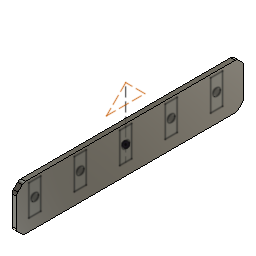
SKADIS_SNS_Label (Autodesk Fusion 360 design; units mm, degrees)
Autodesk Fusion 360 part; units mm, degrees
sketch "SlotLayout" plane through (0, 0, 0) normal (1, 0, 0) x (0, 1, 0)
  line L0 (-22.4, 25) -> (-22.4, 15)
  line L1 (82.4, 5) -> (82.4, -5)
  line L2 (-37.6, -5) -> (-37.6, 5)
  line L3 (-80, 5) -> (-80, -5) construction
  line L4 (-97.6, 15) -> (-97.6, 25)
  line L5 (2.4, -5) -> (2.4, 5)
  arc A0 (-77.6, 5) -> (-82.4, 5) centre (-80, 5) ccw
  arc A1 (22.4, 25) -> (17.6, 25) centre (20, 25) ccw
  arc A2 (-97.6, 25) -> (-102.4, 25) centre (-100, 25) ccw
  arc A3 (97.6, 15) -> (102.4, 15) centre (100, 15) ccw
  line L6 (-60, 25) -> (-60, 15) construction
  line L7 (-77.6, -5) -> (-77.6, 5)
  arc A4 (77.6, -5) -> (82.4, -5) centre (80, -5) ccw
  line L8 (-40, 5) -> (-40, -5) construction
  line L9 (-57.6, 15) -> (-57.6, 25)
  line L10 (-62.4, 25) -> (-62.4, 15)
  line L11 (-102.4, 25) -> (-102.4, 15)
  line L12 (97.6, 15) -> (97.6, 25)
  arc A5 (-102.4, 15) -> (-97.6, 15) centre (-100, 15) ccw
  line L13 (20, 25) -> (20, 15) construction
  line L14 (22.4, 25) -> (22.4, 15)
  line L15 (-80, 0) -> (0, 0) construction
  line L16 (62.4, 25) -> (62.4, 15)
  line L17 (42.4, 5) -> (42.4, -5)
  arc A6 (2.5, 5) -> (-2.5, 5) centre (0, 5) ccw
  arc A7 (2.4, 5) -> (-2.4, 5) centre (0, 5) ccw
  line L18 (80, 5) -> (80, -5) construction
  arc A8 (82.4, 5) -> (77.6, 5) centre (80, 5) ccw
  arc A9 (-2.5, -5) -> (2.5, -5) centre (0, -5) ccw
  arc A10 (57.6, 15) -> (62.4, 15) centre (60, 15) ccw
  arc A11 (62.4, 25) -> (57.6, 25) centre (60, 25) ccw
  line L19 (17.6, 15) -> (17.6, 25)
  line L20 (-20, 25) -> (-20, 15) construction
  line L21 (-42.4, 5) -> (-42.4, -5)
  line L22 (60, 25) -> (60, 15) construction
  arc A12 (42.4, 5) -> (37.6, 5) centre (40, 5) ccw
  line L23 (-100, 25) -> (-100, 15) construction
  line L24 (100, 25) -> (100, 15) construction
  arc A13 (-57.6, 25) -> (-62.4, 25) centre (-60, 25) ccw
  arc A14 (37.6, -5) -> (42.4, -5) centre (40, -5) ccw
  line L25 (40, 5) -> (40, -5) construction
  line L26 (-17.6, 15) -> (-17.6, 25)
  arc A15 (-17.6, 25) -> (-22.4, 25) centre (-20, 25) ccw
  line L27 (-82.4, 5) -> (-82.4, -5)
  line L28 (-2.5, 5) -> (-2.5, -5)
  line L29 (-2.4, 5) -> (-2.4, -5)
  line L30 (102.4, 25) -> (102.4, 15)
  arc A16 (17.6, 15) -> (22.4, 15) centre (20, 15) ccw
  arc A17 (-22.4, 15) -> (-17.6, 15) centre (-20, 15) ccw
  line L31 (37.6, -5) -> (37.6, 5)
  line L32 (0, 5) -> (0, -5) construction
  arc A18 (-62.4, 15) -> (-57.6, 15) centre (-60, 15) ccw
  arc A19 (-42.4, -5) -> (-37.6, -5) centre (-40, -5) ccw
  arc A20 (-2.4, -5) -> (2.4, -5) centre (0, -5) ccw
  arc A21 (102.4, 25) -> (97.6, 25) centre (100, 25) ccw
  arc A22 (-82.4, -5) -> (-77.6, -5) centre (-80, -5) ccw
  arc A23 (-37.6, 5) -> (-42.4, 5) centre (-40, 5) ccw
  line L33 (77.6, -5) -> (77.6, 5)
  line L34 (57.6, 15) -> (57.6, 25)
  line L35 (2.5, -5) -> (2.5, 5)
  point P0 (-20, 20)
  point P1 (-40, 0)
  dimension "d9" = -40
  dimension "d10" = 0
  dimension "d255" = 0.1
  dimension "d22" = 10
  dimension "d23" = 2.4
  dimension "d4" = 40
  dimension "d25" = 40
  dimension "d26" = 20
  dimension "d27" = 20
  constraint tangent L27 A22
  constraint tangent L7 A22
  constraint parallel L7 L27
  constraint tangent A0 L7
  constraint tangent A0 L27
  constraint vertical L3
  constraint tangent L21 A19
  constraint tangent L2 A19
  constraint parallel L2 L21
  constraint tangent L2 A23
  constraint tangent L21 A23
  constraint vertical L8
  constraint tangent L29 A20
  constraint tangent L5 A20
  constraint parallel L5 L29
  constraint tangent L5 A7
  constraint tangent A7 L29
  constraint parallel L2 L32
  constraint midpoint L15.start L3
  constraint midpoint L15.end L32
  constraint horizontal L15
  constraint equal L8 L32
  constraint equal L3 L8
  constraint midpoint P1 L8
  constraint coincident P1 L15
  constraint equal A7 A23
  constraint equal A0 A23
  constraint coincident L15.end origin
  constraint symmetric A0.end L1.start L32
  constraint symmetric L1.end L27.end L32
  constraint symmetric L7.start A4.start L32
  constraint symmetric A8.end A0.start L32
  constraint symmetric A4 L32 A22
  constraint symmetric A0 A8 L32
  constraint symmetric L17.start L21.start L32
  constraint symmetric L17.end L21.end L32
  constraint symmetric A14.start L2.start L32
  constraint symmetric A12.end L2.end L32
  constraint symmetric A14 L32 A19
  constraint symmetric A12 L32 A23
  constraint tangent L0 A17
  constraint tangent L26 A17
  constraint parallel L0 L26
  constraint tangent L26 A15
  constraint tangent L0 A15
  constraint vertical L20
  constraint equal L20 L32
  constraint equal A7 A15
  constraint midpoint P0 L20
  constraint symmetric L0.end L14.end L32
  constraint symmetric L26.end A1.end L32
  constraint symmetric L0.start A1.start L32
  constraint symmetric L26.start L19.start L32
  constraint symmetric A1 A15 L32
  constraint symmetric A16 A17 L32
  constraint symmetric A11.end L9.end L32
  constraint symmetric L16.start L10.start L32
  constraint symmetric A11 A13 L32
  constraint symmetric L16.end L10.end L32
  constraint symmetric A10.start L9.start L32
  constraint symmetric A10 L32 A18
  constraint symmetric L12.end L4.end L32
  constraint symmetric L30.start A2.end L32
  constraint symmetric A2 L32 A21
  constraint symmetric A3.end L11.end L32
  constraint symmetric A3.start L4.start L32
  constraint symmetric A3 A5 L32
  measures "d22" distance of A6.centre A9.centre
  measures "d23" radius of A7
  measures "d4" distance of L8 L32
  measures "d25" distance of L3 L8
  measures "d26" horizontal distance of L20.end A6.centre
  measures "d27" vertical distance of P0 L15.end
sketch "VerticalPrintKey" plane through (0, 0, 0) normal (1, 0, 0) x (0, 1, 0)
  line L0 (-2.6, 6.7) -> (2.6, 6.7)
  line L1 (2.6, 6.7) -> (2.6, -6.7)
  line L2 (2.6, -6.7) -> (-2.6, -6.7)
  line L3 (-2.6, -6.7) -> (-2.6, 6.7)
  line L4 (0, 6.7) -> (0, -6.7) construction
  circle A0 centre (0, 0) radius 1.6
  line L5 (2.6, 0) -> (20.8722, 0) construction
  line L6 (20.8722, 0) -> (11.7361, 9.1361) construction
  line L7 (11.7361, 9.1361) -> (11.7361, -9.1361) construction
  line L8 (11.7361, -9.1361) -> (20.8722, 0) construction
  dimension "d18" = 13.4
  dimension "d19" = 5.2
  dimension "d20" = 3.2
  constraint horizontal L0
  constraint vertical L1
  constraint horizontal L2
  constraint vertical L3
  constraint midpoint L0 L4.start
  constraint midpoint L2 L4.end
  constraint midpoint L4 A0.centre
  constraint coincident A0.centre origin
  constraint midpoint L1 L5.start
  constraint perpendicular L1 L5
  constraint perpendicular L5 L7
  constraint perpendicular L6 L8
  constraint midpoint L5 L7
  measures "d18" distance of L4.start L4.end
  measures "d19" distance of L1 L3
  measures "d20" diameter of A0
sketch "HorizontalPrintKey" plane through (0, 0, 0) normal (1, 0, 0) x (0, 1, 0)
  circle A0 centre (0, 0) radius 1.6
  line L0 (2.6, -6.7) -> (-2.6, -6.7)
  line L1 (-2.6, -6.7) -> (-2.6, 6.7)
  line L2 (-2.6, 6.7) -> (2.6, 6.7)
  line L3 (2.6, 6.7) -> (2.6, -6.7)
  line L4 (0, 6.7) -> (0, -6.7) construction
  line L5 (0, 6.7) -> (0, 23.5939) construction
  line L6 (0, 23.5939) -> (-8.4469, 15.1469) construction
  line L7 (-8.4469, 15.1469) -> (8.4469, 15.1469) construction
  line L8 (8.4469, 15.1469) -> (0, 23.5939) construction
  line L9 (17.4, -6.7) -> (17.4, 6.7)
  line L10 (17.4, 6.7) -> (22.6, 6.7)
  line L11 (22.6, -6.7) -> (17.4, -6.7)
  line L12 (22.6, 6.7) -> (22.6, -6.7)
  circle A1 centre (20, 0) radius 1.6
  line L13 (37.4, -6.7) -> (37.4, 6.7)
  line L14 (37.4, 6.7) -> (42.6, 6.7)
  line L15 (42.6, -6.7) -> (37.4, -6.7)
  line L16 (42.6, 6.7) -> (42.6, -6.7)
  circle A2 centre (40, 0) radius 1.6
  line L17 (-37.4, 6.7) -> (-42.6, 6.7)
  line L18 (-22.6, -6.7) -> (-17.4, -6.7)
  line L19 (-42.6, -6.7) -> (-37.4, -6.7)
  line L20 (-37.4, -6.7) -> (-37.4, 6.7)
  circle A3 centre (-40, 0) radius 1.6
  circle A4 centre (-20, 0) radius 1.6
  line L21 (-42.6, 6.7) -> (-42.6, -6.7)
  line L22 (-22.6, 6.7) -> (-22.6, -6.7)
  line L23 (-17.4, -6.7) -> (-17.4, 6.7)
  line L24 (-17.4, 6.7) -> (-22.6, 6.7)
  dimension "d21" = 13.4
  dimension "d24" = 5.2
  dimension "d28" = 3.2
  dimension "d32" = 20
  dimension "d33" = 0
  constraint horizontal L2
  constraint vertical L3
  constraint horizontal L0
  constraint vertical L1
  constraint midpoint L4.start L2
  constraint midpoint L4.end L0
  constraint midpoint A0.centre L4
  constraint coincident A0.centre origin
  constraint perpendicular L2 L5
  constraint perpendicular L5 L7
  constraint midpoint L5 L7
  constraint perpendicular L6 L8
  constraint symmetric L5 L9.start L18.end
  constraint symmetric L5 L9.end L23.end
  constraint symmetric L5 L10.end L22.start
  constraint symmetric L5 L11.start L18.start
  constraint symmetric L5 A1 A4
  constraint symmetric L5 L13.start L19.end
  constraint symmetric L5 L13.end L17.start
  constraint symmetric L5 L14.end L17.end
  constraint symmetric L5 L15.start L19.start
  constraint symmetric L5 A2 A3
  measures "d21" distance of L4.end L4.start
  measures "d24" distance of L1 L3
  measures "d28" diameter of A0
sketch "Sketch1" plane through (0, 0, 0) normal (1, 0, 0) x (0, 1, 0) in component "LabelMount_100"
  line L0 (-50, 10) -> (50, 10)
  line L1 (50, 10) -> (50, -10)
  line L2 (50, -10) -> (-50, -10)
  line L3 (-50, -10) -> (-50, 10)
  line L4 (-50, 0) -> (50, 0) construction
  line L5 (0, 10) -> (0, -10) construction
  dimension "d34" = 20
  dimension "d35" = 100
  constraint horizontal L0
  constraint vertical L1
  constraint horizontal L2
  constraint vertical L3
  constraint midpoint L3 L4.start
  constraint midpoint L1 L4.end
  constraint midpoint L0 L5.start
  constraint midpoint L2 L5.end
  constraint midpoint L5 origin
  measures "d34" distance of L0.start L2.end
  measures "d35" distance of L4.start L4.end
extrude "Extrude1" add sketch "Sketch1" along normal blind 2 makes body 1 in component "LabelMount_100"
extrude "Extrude2" cut sketch "HorizontalPrintKey" along normal blind 1.2 contours A0 | L0 L1 L2 L3 | L9 L10 L11 L12 | A1 | L13 L14 L15 L16 | A2 | L17 L19 L20 L21 | L18 L22 L23 L24 | A3 | A4 bodies 1 in component "LabelMount_100"
chamfer "Chamfer1" distance 3 angle 45 4 edges at (1, -50, 10) (1, -50, -10) (1, 50, 10) (1, 50, -10) on bodies 1 in component "LabelMount_100"
fillet "Fillet1" radius 2 8 edges at (1, -50, 7) (1, -47, 10) (1, -50, -7) (1, -47, -10) (1, 47, 10) (1, 50, 7) (1, 50, -7) (1, 47, -10) on bodies 1 in component "LabelMount_100"
sketch "Sketch1 (2)" plane through (0, 0, 0) normal (1, 0, 0) x (0, 1, 0) in component "LabelMount_80"
  line L0 (-50, 10) -> (50, 10)
  line L1 (50, 10) -> (50, -10)
  line L2 (50, -10) -> (-50, -10)
  line L3 (-50, -10) -> (-50, 10)
  line L4 (-50, 0) -> (50, 0) construction
  line L5 (0, 10) -> (0, -10) construction
  line L6 (30, 10) -> (30, -10)
  dimension "d34_1" = 20
  dimension "d35_1" = 100
  dimension "d43" = 80
  constraint horizontal L0
  constraint vertical L1
  constraint horizontal L2
  constraint vertical L3
  constraint midpoint L3 L4.start
  constraint midpoint L1 L4.end
  constraint midpoint L0 L5.start
  constraint midpoint L2 L5.end
  constraint midpoint L5 origin
  constraint coincident L0 L6.start
  constraint coincident L2 L6.end
  constraint perpendicular L2 L6
  measures "d34_1" distance of L0.start L2.end
  measures "d35_1" distance of L4.start L4.end
  measures "d43" distance of L3 L6
extrude "Extrude1'" add sketch "Sketch1 (2)" along normal blind 2 separate body contours L0 L2 L3 L6 makes body 2 in component "LabelMount_80"
extrude "Extrude2'" cut sketch "HorizontalPrintKey" along normal blind 1.2 contours A0 | L0 L1 L2 L3 | L9 L10 L11 L12 | A1 | L13 L14 L15 L16 | A2 | L17 L19 L20 L21 | L18 L22 L23 L24 | A3 | A4 bodies 2 in component "LabelMount_80"
chamfer "Chamfer1'" distance 3 angle 45 4 edges at (1, -50, 10) (1, -50, -10) (1, 30, 10) (1, 30, -10) on bodies 2 in component "LabelMount_80"
fillet "Fillet1'" radius 2 8 edges at (1, -50, 7) (1, -47, 10) (1, -50, -7) (1, -47, -10) (1, 27, 10) (1, 30, 7) (1, 30, -7) (1, 27, -10) on bodies 2 in component "LabelMount_80"
sketch "Sketch1 (3)" plane through (0, 0, 0) normal (1, 0, 0) x (0, 1, 0) in component "LabelMount_60"
  line L0 (-50, 10) -> (50, 10)
  line L1 (50, 10) -> (50, -10)
  line L2 (50, -10) -> (-50, -10)
  line L3 (-50, -10) -> (-50, 10)
  line L4 (-50, 0) -> (50, 0) construction
  line L5 (0, 10) -> (0, -10) construction
  line L6 (10, 10) -> (10, -10)
  dimension "d34_1_1" = 20
  dimension "d35_1_1" = 100
  dimension "d43_1" = 60
  constraint horizontal L0
  constraint vertical L1
  constraint horizontal L2
  constraint vertical L3
  constraint midpoint L3 L4.start
  constraint midpoint L1 L4.end
  constraint midpoint L0 L5.start
  constraint midpoint L2 L5.end
  constraint midpoint L5 origin
  constraint coincident L0 L6.start
  constraint coincident L2 L6.end
  constraint perpendicular L2 L6
  measures "d34_1_1" distance of L0.start L2.end
  measures "d35_1_1" distance of L4.start L4.end
  measures "d43_1" distance of L3 L6
extrude "Extrude1''" add sketch "Sketch1 (3)" along normal blind 2 separate body contours L0 L2 L3 L6 makes body 3 in component "LabelMount_60"
extrude "Extrude2''" cut sketch "HorizontalPrintKey" along normal blind 1.2 contours A0 | L0 L1 L2 L3 | L9 L10 L11 L12 | A1 | L13 L14 L15 L16 | A2 | L17 L19 L20 L21 | L18 L22 L23 L24 | A3 | A4 bodies 3 in component "LabelMount_60"
chamfer "Chamfer1''" distance 3 angle 45 4 edges at (1, -50, 10) (1, -50, -10) (1, 10, 10) (1, 10, -10) on bodies 3 in component "LabelMount_60"
fillet "Fillet1''" radius 2 8 edges at (1, -50, 7) (1, -47, 10) (1, -50, -7) (1, -47, -10) (1, 7, 10) (1, 10, 7) (1, 10, -7) (1, 7, -10) on bodies 3 in component "LabelMount_60"
sketch "Sketch1 (4)" plane through (0, 0, 0) normal (1, 0, 0) x (0, 1, 0) in component "LabelMount_40"
  line L0 (-50, 10) -> (50, 10)
  line L1 (50, 10) -> (50, -10)
  line L2 (50, -10) -> (-50, -10)
  line L3 (-50, -10) -> (-50, 10)
  line L4 (-50, 0) -> (50, 0) construction
  line L5 (0, 10) -> (0, -10) construction
  line L6 (-10, 10) -> (-10, -10)
  dimension "d34_1_1_1" = 20
  dimension "d35_1_1_1" = 100
  dimension "d43_1_1" = 40
  constraint horizontal L0
  constraint vertical L1
  constraint horizontal L2
  constraint vertical L3
  constraint midpoint L3 L4.start
  constraint midpoint L1 L4.end
  constraint midpoint L0 L5.start
  constraint midpoint L2 L5.end
  constraint midpoint L5 origin
  constraint coincident L0 L6.start
  constraint coincident L2 L6.end
  constraint perpendicular L2 L6
  measures "d34_1_1_1" distance of L0.start L2.end
  measures "d35_1_1_1" distance of L4.start L4.end
  measures "d43_1_1" distance of L3 L6
extrude "Extrude1'''" add sketch "Sketch1 (4)" along normal blind 2 separate body contours L0 L2 L3 L6 makes body 4 in component "LabelMount_40"
extrude "Extrude2'''" cut sketch "HorizontalPrintKey" along normal blind 1.2 contours A0 | L0 L1 L2 L3 | L9 L10 L11 L12 | A1 | L13 L14 L15 L16 | A2 | L17 L19 L20 L21 | L18 L22 L23 L24 | A3 | A4 bodies 4 in component "LabelMount_40"
chamfer "Chamfer1'''" distance 3 angle 45 4 edges at (1, -50, 10) (1, -50, -10) (1, -10, 10) (1, -10, -10) on bodies 4 in component "LabelMount_40"
fillet "Fillet1'''" radius 2 8 edges at (1, -50, 7) (1, -47, 10) (1, -50, -7) (1, -47, -10) (1, -13, 10) (1, -10, 7) (1, -10, -7) (1, -13, -10) on bodies 4 in component "LabelMount_40"
component "LabelMount_100" placed x (1, 0, 0) y (0, 1, 0) z (0, 0, 1) at (0, 0, 0)
component "LabelMount_80" placed x (1, 0, 0) y (0, 1, 0) z (0, 0, 1) at (0, 0, 0)
component "LabelMount_60" placed x (1, 0, 0) y (0, 1, 0) z (0, 0, 1) at (0, 0, 0)
component "LabelMount_40" placed x (1, 0, 0) y (0, 1, 0) z (0, 0, 1) at (0, 0, 0)
equation "XY_Tolerance = 0.2 mm"
equation "Z_Tolerance = 0.2 mm"
equation "Wall_Thickness = 0.4 mm"
equation "Layer_Height = 0.2 mm"
equation "M3Hole_wClearance = 3.2 mm"
equation "M3Hole_wSelfTapping = 2.8 mm"
equation "d20 = M3Hole_wClearance"
equation "d28 = M3Hole_wClearance"
equation "M3Hole_CounterSink = 1.8 mm"
named bodies: "LabeMount_100", "LabelMount_80", "LabelMount_60", "LabelMount_40"
